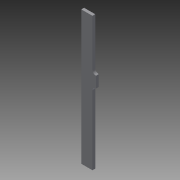
# Autodesk Inventor part: Granny Gearbox Routing Template Vertical Tabs
Saved by Autodesk Inventor 2015 (Build 190159000, 159)
## iProperties
Created: 2016-02-25
Part Number: Granny Gearbox Routing Template Vertical Tabs
Material: Generic
Document SubType Name: Modeling
Designer: sethbattis
Density: 1 g/cm^3
Appearance: Default
Author: sethbattis
Autodesk Inventor part; units mm, degrees
ref_plane "YZ Plane" through (0, 0, 0) normal (1, 0, 0) x (0, 1, 0)
ref_plane "XZ Plane" through (0, 0, 0) normal (0, 1, 0) x (-1, 0, 0)
ref_plane "XY Plane" through (0, 0, 0) normal (0, 0, 1) x (1, 0, 0)
sketch "Sketch1" plane through (0, 0, 0) normal (0, 0, 1) x (1, 0, 0)
  line L0 (-4.0353, 2.9403) -> (8.6647, 2.9403)
  line L1 (8.6647, 2.9403) -> (8.6647, -50.241)
  line L2 (8.6647, -149.4597) -> (-4.0353, -149.4597)
  line L3 (-4.0353, -149.4597) -> (-4.0353, 2.9403)
  line L4 (12.6335, -54.2097) -> (12.6335, -54.2097)
  line L5 (12.6335, -54.2097) -> (12.6335, -66.9097)
  line L6 (12.6335, -66.9097) -> (12.6335, -66.9097)
  line L7 (8.6647, -70.8785) -> (8.6647, -149.4597)
  arc A0 (8.6647, -50.241) -> (12.6335, -54.2097) centre (12.6335, -50.241) ccw
  arc A1 (12.6335, -66.9097) -> (8.6647, -70.8785) centre (12.6335, -70.8785) ccw
  point P0 (0, 0)
  point P1 (8.6647, -66.9097)
  dimension "d0" = 12.7
  dimension "d1" = 152.4
  dimension "d2" = 3.9688
  dimension "d3" = 12.7
  dimension "d4" = 3.9688
  dimension "d5" = 57.15
  constraints: 16 end point, 4 parallel, 4 point on circle, 4 tangent, 3 perpendicular, 2 centre point, 2 horizontal, 2 point on line, 1 equal radius
  measures "d0" distance of L2.start L2.end
  measures "d1" distance of L0.end L2.start
  measures "d2" distance of L5.end point (8.665, -66.91)
  measures "d3" distance of L4.end L5.end
  measures "d4" radius of A0
  measures "d5" distance from line of L4.end L0
extrude "Extrusion1" add sketch "Sketch1" along normal blind 3.175
body "Solid1"
